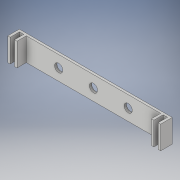
# Autodesk Inventor part: Potentiometer Carrier
Saved by Autodesk Inventor 2019 (Build 230136000, 136)
## iProperties
Created: 2019-01-04
Part Number: Potentiometer Carrier
Material: Generic
Document SubType Name: Modeling
Designer: Martin
Density: 1 g/cm^3
Appearance: Default
Author: Martin
Autodesk Inventor part; units mm, degrees
note: some values were not read from the file. Chosen so that the rebuilt part matches the saved one: direction of "Emboss1".
ref_plane "YZ Plane" through (0, 0, 0) normal (1, 0, 0) x (0, 1, 0)
ref_plane "XZ Plane" through (0, 0, 0) normal (0, 1, 0) x (-1, 0, 0)
ref_plane "XY Plane" through (0, 0, 0) normal (0, 0, 1) x (1, 0, 0)
sketch "Sketch1" plane through (0, 0, 0) normal (0, 0, 1) x (1, 0, 0)
  line L0 (-66, 10) -> (66, 10)
  line L1 (66, 10) -> (66, -10)
  line L2 (66, -10) -> (-66, -10)
  line L3 (-66, -10) -> (-66, 10)
  line L4 (-63.85, 10) -> (63.85, 10) construction
  line L5 (63.85, 10) -> (63.85, -10) construction
  line L6 (63.85, -10) -> (-63.85, -10) construction
  line L7 (-63.85, -10) -> (-63.85, 10) construction
  line L8 (-60.15, 10) -> (60.15, 10) construction
  line L9 (60.15, 10) -> (60.15, -10) construction
  line L10 (60.15, -10) -> (-60.15, -10) construction
  line L11 (-60.15, -10) -> (-60.15, 10) construction
  line L12 (-58, 10) -> (58, 10) construction
  line L13 (58, 10) -> (58, -10) construction
  line L14 (58, -10) -> (-58, -10) construction
  line L15 (-58, -10) -> (-58, 10) construction
  line L16 (-66, 10) -> (-63.85, 10)
  line L17 (-63.85, 10) -> (-63.85, -10)
  line L18 (-63.85, -10) -> (-66, -10)
  line L19 (-66, -10) -> (-66, 10)
  line L20 (-60.15, 10) -> (-58, 10)
  line L21 (-58, 10) -> (-58, -10)
  line L22 (-58, -10) -> (-60.15, -10)
  line L23 (-60.15, -10) -> (-60.15, 10)
  line L24 (58, 10) -> (60.15, 10)
  line L25 (60.15, 10) -> (60.15, -10)
  line L26 (60.15, -10) -> (58, -10)
  line L27 (58, -10) -> (58, 10)
  line L28 (63.85, 10) -> (66, 10)
  line L29 (66, 10) -> (66, -10)
  line L30 (66, -10) -> (63.85, -10)
  line L31 (63.85, -10) -> (63.85, 10)
  dimension "d0" = 132
  dimension "d7" = 20
  dimension "d10" = 2.15
  dimension "d11" = 8
  dimension "d12" = 2.15
  dimension "d13" = 8
  dimension "d14" = 2.15
  dimension "d15" = 2.15
  constraints: 64 end point, 16 parallel, 8 horizontal, 8 perpendicular
  measures "d0" distance of L1.end L2.end
  measures "d7" distance of L12.end L13.end
  measures "d10" distance between parallel lines of L17 L3
  measures "d11" distance between parallel lines of L15 L3
  measures "d12" distance between parallel lines of L11 L21
  measures "d13" distance between parallel lines of L13 L1
  measures "d14" distance between parallel lines of L1 L5
  measures "d15" distance between parallel lines of L9 L13
extrude "Extrusion1" add sketch "Sketch1" against normal blind 2
extrude "Extrusion2" add sketch "Sketch1" along normal blind 8 contours L0 L17 L2 L3 | L0 L21 L2 L23 | L0 L25 L2 L27 | L0 L1 L2 L31
sketch "Sketch2" plane through (0, 0, -2) normal (0, 0, -1) x (-1, 0, 0)
  line L0 (0, 19.4414) -> (0, -19.8832)
  circle A0 centre (0, 0) radius 3.55
  circle A1 centre (-30, 0) radius 3.55
  circle A2 centre (30, 0) radius 3.55
  dimension "d18" = 7.1
  dimension "d19" = 7.1
  dimension "d20" = 30
  constraints: 3 centre point, 2 end point, 1 coincident, 1 symmetric about line, 1 vertical, 1 other
  measures "d18" diameter of A0
  measures "d19" diameter of A1
  measures "d20" distance of A1.centre point (0, 0)
extrude "Extrusion3" cut sketch "Sketch2" against normal blind 8
sketch "Sketch3" plane through (0, 0, -2) normal (0, 0, -1) x (-1, 0, 0)
  line L0 (-31.3557, -7) -> (-28.645, -7) construction
  line L1 (-28.645, -7) -> (-28.645, -7.465) construction
  line L2 (-28.645, -7.465) -> (-31.3557, -7.465) construction
  line L3 (-31.3557, -7.465) -> (-31.3557, -7) construction
  line L4 (-68.5578, -7) -> (66.8364, -7) construction
  line L5 (-66, -10) -> (66, -10) construction
  line L6 (-0.6824, -6.1354) -> (0.8811, -6.1354) construction
  line L7 (0.8811, -6.1354) -> (0.8811, -8.5213) construction
  line L8 (0.8811, -8.5213) -> (-0.6824, -8.5213) construction
  line L9 (-0.6824, -8.5213) -> (-0.6824, -6.1354) construction
  line L10 (29.0008, -5.8043) -> (31.8438, -5.8043) construction
  line L11 (31.8438, -5.8043) -> (31.8438, -8.8523) construction
  line L12 (31.8438, -8.8523) -> (29.0008, -8.8523) construction
  line L13 (29.0008, -8.8523) -> (29.0008, -5.8043) construction
  line L14 (-66.6378, -5.8043) -> (67.7633, -5.8043) construction
  spline S0 degree 2 poles (-28.7374, -6.6782) (-28.7374, -6.8873) (-28.8711, -7.2665) (-28.9951, -7.3929) knots 0 0 0 1 2 2 2
  spline S1 degree 2 poles (-28.9951, -7.3929) (-29.0704, -7.4732) (-29.2552, -7.6044) (-29.3646, -7.6506) knots 0 0 0 1 2 2 2
  spline S2 degree 2 poles (-29.3646, -7.6506) (-29.4764, -7.6968) (-29.7366, -7.7503) (-29.897, -7.7503) knots 0 0 0 1 2 2 2
  line L15 (-29.897, -7.7503) -> (-30.2909, -7.7503)
  line L16 (-30.2909, -7.7503) -> (-30.2909, -8.7325)
  line L17 (-30.2909, -8.7325) -> (-31.0445, -8.7325)
  line L18 (-31.0445, -8.7325) -> (-31.0445, -5.7325)
  line L19 (-31.0445, -5.7325) -> (-29.88, -5.7325)
  spline S3 degree 2 poles (-29.88, -5.7325) (-29.6223, -5.7325) (-29.2455, -5.8273) (-29.0923, -5.9294) knots 0 0 0 1 2 2 2
  spline S4 degree 2 poles (-29.0923, -5.9294) (-28.9221, -6.0437) (-28.7374, -6.4181) (-28.7374, -6.6782) knots 0 0 0 1 2 2 2
  spline S5 degree 2 poles (-29.5105, -6.6976) (-29.5105, -6.5688) (-29.632, -6.3865) (-29.7147, -6.3524) knots 0 0 0 1 2 2 2
  spline S6 degree 2 poles (-29.7147, -6.3524) (-29.8217, -6.3062) (-30.0162, -6.2916) (-30.1839, -6.2916) knots 0 0 0 1 2 2 2
  line L20 (-30.1839, -6.2916) -> (-30.2909, -6.2916)
  line L21 (-30.2909, -6.2916) -> (-30.2909, -7.1912)
  line L22 (-30.2909, -7.1912) -> (-30.2374, -7.1912)
  spline S7 degree 2 poles (-30.2374, -7.1912) (-30.1328, -7.1912) (-29.9432, -7.1863) (-29.8727, -7.1741) knots 0 0 0 1 2 2 2
  spline S8 degree 2 poles (-29.8727, -7.1741) (-29.8119, -7.1644) (-29.6782, -7.1061) (-29.6418, -7.0696) knots 0 0 0 1 2 2 2
  spline S9 degree 2 poles (-29.6418, -7.0696) (-29.564, -6.9967) (-29.5105, -6.8338) (-29.5105, -6.6976) knots 0 0 0 1 2 2 2
  line L23 (0.9064, -8.8283) -> (-0.7078, -8.8283)
  line L24 (-0.7078, -8.8283) -> (-0.7078, -8.3056)
  line L25 (-0.7078, -8.3056) -> (-0.2775, -8.3056)
  line L26 (-0.2775, -8.3056) -> (-0.2775, -6.351)
  line L27 (-0.2775, -6.351) -> (-0.7078, -6.351)
  line L28 (-0.7078, -6.351) -> (-0.7078, -5.8283)
  line L29 (-0.7078, -5.8283) -> (0.9064, -5.8283)
  line L30 (0.9064, -5.8283) -> (0.9064, -6.351)
  line L31 (0.9064, -6.351) -> (0.4761, -6.351)
  line L32 (0.4761, -6.351) -> (0.4761, -8.3056)
  line L33 (0.4761, -8.3056) -> (0.9064, -8.3056)
  line L34 (0.9064, -8.3056) -> (0.9064, -8.8283)
  spline S10 degree 2 poles (31.8482, -7.3307) (31.8482, -7.7513) (31.4811, -8.4126) (31.2015, -8.5901) knots 0 0 0 1 2 2 2
  spline S11 degree 2 poles (31.2015, -8.5901) (30.9681, -8.7408) (30.4187, -8.8283) (30.1099, -8.8283) knots 0 0 0 1 2 2 2
  line L35 (30.1099, -8.8283) -> (29.1715, -8.8283)
  line L36 (29.1715, -8.8283) -> (29.1715, -5.8283)
  line L37 (29.1715, -5.8283) -> (30.1002, -5.8283)
  spline S12 degree 2 poles (30.1002, -5.8283) (30.4162, -5.8283) (30.9681, -5.9085) (31.2112, -6.0641) knots 0 0 0 1 2 2 2
  spline S13 degree 2 poles (31.2112, -6.0641) (31.5054, -6.2538) (31.8482, -6.8956) (31.8482, -7.3307) knots 0 0 0 1 2 2 2
  spline S14 degree 2 poles (31.0751, -7.3259) (31.0751, -7.0293) (30.8709, -6.6063) (30.6618, -6.4872) knots 0 0 0 1 2 2 2
  spline S15 degree 2 poles (30.6618, -6.4872) (30.5086, -6.4045) (30.1731, -6.3875) (29.9397, -6.3875) knots 0 0 0 1 2 2 2
  line L38 (29.9397, -6.3875) -> (29.9251, -6.3875)
  line L39 (29.9251, -6.3875) -> (29.9251, -8.2667)
  line L40 (29.9251, -8.2667) -> (29.9397, -8.2667)
  spline S16 degree 2 poles (29.9397, -8.2667) (30.1926, -8.2667) (30.5402, -8.2497) (30.6982, -8.15) knots 0 0 0 1 2 2 2
  spline S17 degree 2 poles (30.6982, -8.15) (30.883, -8.0333) (31.0751, -7.6225) (31.0751, -7.3259) knots 0 0 0 1 2 2 2
  point P0 (0, 0)
  dimension "d23" = 28.645
  dimension "d24" = 2.7107
  dimension "d25" = 3
  constraints: 4 end point, 2 horizontal, 1 collinear, 6 other
  measures "d23" horizontal distance of point (0, 0) L1.end
  measures "d24" distance between parallel lines of L1 L3
  measures "d25" distance between parallel lines of L4 L5
emboss "Emboss1" sketch "Sketch3" operation cut depth 1 direction (0, 0, 1)
body "Solid1"
